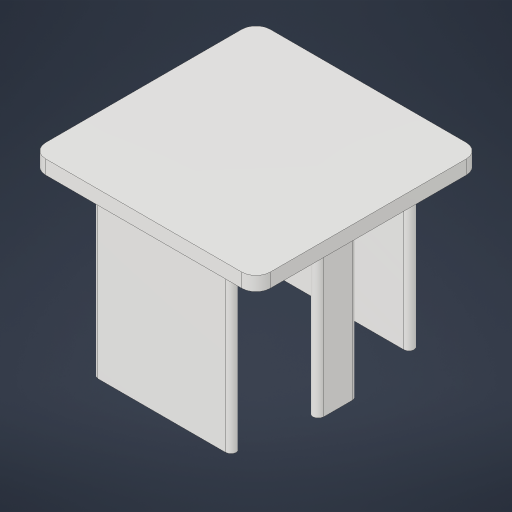
# Autodesk Inventor part: vrm tool
Saved by Autodesk Inventor 2023.4 (Build 274418000, 418)
## iProperties
Created: 2025-02-18
Part Number: vrm tool
Material: ABS Plastic
Document SubType Name: Modeling
Designer: brand
Density: 1.06 g/cm^3
Appearance: Smooth - White
Author: brand
Autodesk Inventor part; units mm, degrees
ref_plane "YZ Plane" through (0, 0, 0) normal (1, 0, 0) x (0, 1, 0)
ref_plane "XZ Plane" through (0, 0, 0) normal (0, 1, 0) x (-1, 0, 0)
ref_plane "XY Plane" through (0, 0, 0) normal (0, 0, 1) x (1, 0, 0)
sketch "Sketch1" plane through (0, 0, 0) normal (0, 1, 0) x (-1, 0, 0)
  line L0 (15.875, 20.1549) -> (-15.875, 20.1549) construction
  line L1 (14.478, 18.7579) -> (-14.478, 18.7579) construction
  line L2 (-14.478, 21.5519) -> (14.478, 21.5519) construction
  arc A0 (14.478, 18.7579) -> (14.478, 21.5519) centre (14.478, 20.1549) ccw construction
  arc A1 (-14.478, 21.5519) -> (-14.478, 18.7579) centre (-14.478, 20.1549) ccw construction
  line L3 (25.4, -25.4) -> (-25.4, -25.4)
  line L4 (-25.4, -25.4) -> (-25.4, 25.4)
  line L5 (-25.4, 25.4) -> (25.4, 25.4)
  line L6 (25.4, 25.4) -> (25.4, -25.4)
  line L7 (25.4, -25.4) -> (-25.4, 25.4) construction
  line L8 (-25.4, -25.4) -> (25.4, 25.4) construction
  line L9 (-15.875, -20.1549) -> (15.875, -20.1549) construction
  line L10 (-14.478, -18.7579) -> (14.478, -18.7579) construction
  line L11 (14.478, -21.5519) -> (-14.478, -21.5519) construction
  arc A2 (-14.478, -18.7579) -> (-14.478, -21.5519) centre (-14.478, -20.1549) ccw construction
  arc A3 (14.478, -21.5519) -> (14.478, -18.7579) centre (14.478, -20.1549) ccw construction
  line L12 (0, -20.1549) -> (0, 20.1549) construction
  line L13 (-17.3355, -4.699) -> (-17.3355, 4.699) construction
  line L14 (-15.875, -3.2385) -> (-15.875, 3.2385) construction
  line L15 (-18.796, 3.2385) -> (-18.796, -3.2385) construction
  arc A4 (-18.796, -3.2385) -> (-15.875, -3.2385) centre (-17.3355, -3.2385) ccw construction
  arc A5 (-15.875, 3.2385) -> (-18.796, 3.2385) centre (-17.3355, 3.2385) ccw construction
  line L16 (-14.478, -21.2979) -> (14.478, -21.2979)
  arc A6 (14.478, -21.2979) -> (14.478, -19.0119) centre (14.478, -20.1549) ccw
  line L17 (14.478, -19.0119) -> (-14.478, -19.0119)
  arc A7 (-14.478, -19.0119) -> (-14.478, -21.2979) centre (-14.478, -20.1549) ccw
  line L18 (-14.478, 19.0119) -> (14.478, 19.0119)
  arc A8 (14.478, 19.0119) -> (14.478, 21.2979) centre (14.478, 20.1549) ccw
  line L19 (14.478, 21.2979) -> (-14.478, 21.2979)
  arc A9 (-14.478, 21.2979) -> (-14.478, 19.0119) centre (-14.478, 20.1549) ccw
  line L20 (-16.129, 3.2385) -> (-16.129, -3.2385)
  arc A10 (-18.542, -3.2385) -> (-16.129, -3.2385) centre (-17.3355, -3.2385) ccw
  line L21 (-18.542, -3.2385) -> (-18.542, 3.2385)
  arc A11 (-16.129, 3.2385) -> (-18.542, 3.2385) centre (-17.3355, 3.2385) ccw
  point P0 (0, 0)
  point P1 (0, 0)
  point P2 (-17.3355, 0)
  point P3 (-15.875, -20.1549)
  dimension "d0" = 31.75
  dimension "d1" = 50.8
  dimension "d2" = 50.8
  dimension "d3" = 37.5158
  dimension "d4" = 2.794
  dimension "d5" = 31.75
  dimension "d6" = 2.794
  dimension "d7" = 9.398
  dimension "d8" = 2.921
  dimension "clear" = 0.254
  dimension "d10" = 0.254
  dimension "d11" = 0.254
  constraints: 50 end point, 33 point on circle, 12 centre point, 12 tangent, 8 parallel, 6 midpoint, 6 point on line, 3 horizontal, 3 vertical alignment, 2 perpendicular, 1 coincident, 1 horizontal alignment, 1 vertical, 9 other
  measures "d0" distance of point (-15.875, 20.155) point (15.875, 20.155)
  measures "d1" distance of L3.start L3.end
  measures "d2" distance of L3.end L4.end
  measures "d3" distance between parallel lines of L1 L10
  measures "d4" distance between parallel lines of L2 L1
  measures "d5" distance of L9.start L9.end
  measures "d6" distance between parallel lines of L11 L10
  measures "d7" distance of L13.start L13.end
  measures "d8" distance between parallel lines of L14 L15
  measures "clear" distance between parallel lines of L11 L16
  measures "d10" distance between parallel lines of L1 L18
  measures "d11" distance between parallel lines of L14 L20
extrude "Extrusion1" add sketch "Sketch1" along normal blind 3.175 contours L3 L4 L5 L6 | A7 L17 A6 L16 | A9 L19 A8 L18 | L20 A10 L21 A11
extrude "Extrusion2" add sketch "Sketch1" against normal blind 38.1 contours A7 L17 A6 L16 | A9 L19 A8 L18 | L20 A10 L21 A11
fillet "Fillet1" radius 3.175 4 edges at (25.4, 1.5875, 25.4) (-25.4, 1.5875, 25.4) (25.4, 1.5875, -25.4) (-25.4, 1.5875, -25.4)
fillet "Fillet2" radius 3.175 12 edges at (0, 0, -21.2979) (-15.621, 0, -20.1549) (0, 0, -19.0119) (15.621, 0, -20.1549) (17.3355, 0, 4.445) (18.542, 0, 0) (17.3355, 0, -4.445) (16.129, 0, 0) (-15.621, 0, 20.1549) (0, 0, 21.2979) (15.621, 0, 20.1549) (0, 0, 19.0119)
equation "\"d5\" = d0"
equation "\"d6\" = d4"
equation "\"d10\" = clear"
equation "\"d11\" = clear"
body "Solid1"
